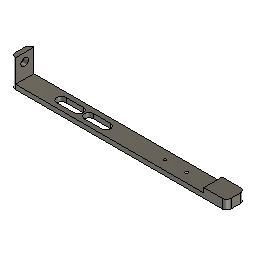
gearmotor winding v0 (Autodesk Fusion 360 design; units mm, degrees)
Autodesk Fusion 360 part; units mm, degrees
sketch "Sketch1" plane through (0, 0, 0) normal (0, 0, 1) x (1, 0, 0)
  line L0 (-70, 20) -> (165, 20)
  line L1 (165, 20) -> (165, 0)
  line L2 (165, 0) -> (-70, 0)
  line L3 (-70, 0) -> (-70, 20)
  dimension "d1" = 235
  dimension "d2" = 20
  constraint horizontal L0
  constraint vertical L1
  constraint horizontal L2
  constraint vertical L3
  measures "d1" distance of L0.start L0.end
  measures "d2" distance of L0.start L2.end
extrude "Extrude1" add sketch "Sketch1" along normal blind 5
sketch "Sketch2" plane through (0, 0, 5) normal (0, 0, 1) x (-1, 0, 0)
  line L0 (70, 0) -> (-165, 0)
  line L1 (-165, 0) -> (-165, -20)
  line L2 (-165, -20) -> (70, -20)
  line L3 (70, -20) -> (70, 0)
  circle A0 centre (-87.5581, -10.1163) radius 2.5
  circle A1 centre (-111.2788, -10.1163) radius 2.5
  line L4 (25.0313, -5.0352) -> (6.1177, -5.0352)
  arc A2 (6.1177, -5.0352) -> (6.1177, -15.0352) centre (6.1177, -10.0352) ccw
  line L5 (6.1177, -15.0352) -> (25.0313, -15.0352)
  arc A3 (25.0313, -15.0352) -> (25.0313, -5.0352) centre (25.0313, -10.0352) ccw
  line L6 (25.0313, -10.0352) -> (6.1177, -10.0352) construction
  line L7 (-5.3429, -4.8835) -> (-23.6696, -4.8835)
  arc A4 (-23.6696, -4.8835) -> (-23.6696, -14.8835) centre (-23.6696, -9.8835) ccw
  line L8 (-23.6696, -14.8835) -> (-5.3429, -14.8835)
  arc A5 (-5.3429, -14.8835) -> (-5.3429, -4.8835) centre (-5.3429, -9.8835) ccw
  line L9 (-5.3429, -9.8835) -> (-23.6696, -9.8835) construction
  point P0 (6.1177, -10.0352)
  dimension "d5" = 5
  dimension "d6" = 5
  dimension "d7" = 10
  dimension "d8" = 10
  constraint tangent L4 A2
  constraint tangent A2 L5
  constraint parallel L4 L5
  constraint tangent L5 A3
  constraint tangent L4 A3
  constraint parallel L2 L6
  constraint tangent L7 A4
  constraint tangent A4 L8
  constraint parallel L7 L8
  constraint tangent L8 A5
  constraint tangent L7 A5
  constraint parallel L5 L9
  measures "d5" diameter of A0
  measures "d6" diameter of A1
  measures "d7" diameter of A2
  measures "d8" diameter of A4
extrude "Extrude2" cut sketch "Sketch2" against normal blind 20 contours A0 | A1 | L4 A2 L5 A3 | L7 A4 L8 A5
fillet "Fillet1" radius 5 4 edges at (165, 0, 2.5) (165, 20, 2.5) (-70, 20, 2.5) (-70, 0, 2.5)
sketch "Sketch3" plane through (0, 0, 5) normal (0, 0, 1) x (-1, 0, 0)
  arc A0 (70, -5) -> (65, 0) centre (65, -5) ccw
  line L0 (65, 0) -> (-160, 0)
  arc A1 (-160, 0) -> (-165, -5) centre (-160, -5) ccw
  line L1 (-165, -5) -> (-165, -15)
  arc A2 (-165, -15) -> (-160, -20) centre (-160, -15) ccw
  line L2 (-160, -20) -> (65, -20)
  arc A3 (65, -20) -> (70, -15) centre (65, -15) ccw
  line L3 (70, -15) -> (70, -5)
  line L4 (6.1177, -5.0352) -> (25.0313, -5.0352)
  arc A4 (25.0313, -15.0352) -> (25.0313, -5.0352) centre (25.0313, -10.0352) ccw
  line L5 (25.0313, -15.0352) -> (6.1177, -15.0352)
  arc A5 (6.1177, -5.0352) -> (6.1177, -15.0352) centre (6.1177, -10.0352) ccw
  circle A6 centre (-111.2788, -10.1163) radius 2.5
  line L6 (-23.6696, -4.8835) -> (-5.3429, -4.8835)
  arc A7 (-5.3429, -14.8835) -> (-5.3429, -4.8835) centre (-5.3429, -9.8835) ccw
  line L7 (-5.3429, -14.8835) -> (-23.6696, -14.8835)
  arc A8 (-23.6696, -4.8835) -> (-23.6696, -14.8835) centre (-23.6696, -9.8835) ccw
  circle A9 centre (-87.5581, -10.1163) radius 2.5
  line L8 (-165, -20) -> (-140, -20)
  line L9 (-140, -20) -> (-140, 0)
  line L10 (-140, 0) -> (-165, 0)
  line L11 (-165, 0) -> (-165, -20)
  dimension "d13" = 25
  dimension "d14" = 20
  constraint horizontal L8
  constraint vertical L9
  constraint horizontal L10
  constraint vertical L11
  measures "d13" distance of L8.start L8.end
  measures "d14" distance of L8.start L10.end
extrude "Extrude3" add sketch "Sketch3" along normal blind 5 contours L0 A1 L1 A2 L2 L8 L9 L10 L11
sketch "Sketch4" plane through (0, 0, 5) normal (0, 0, 1) x (-1, 0, 0)
  line L0 (-140, 0) -> (-140, -20)
  line L1 (-140, -20) -> (65, -20)
  arc A0 (65, -20) -> (70, -15) centre (65, -15) ccw
  line L2 (70, -15) -> (70, -5)
  arc A1 (70, -5) -> (65, 0) centre (65, -5) ccw
  line L3 (65, 0) -> (-140, 0)
  line L4 (6.1177, -5.0352) -> (25.0313, -5.0352)
  arc A2 (25.0313, -15.0352) -> (25.0313, -5.0352) centre (25.0313, -10.0352) ccw
  line L5 (25.0313, -15.0352) -> (6.1177, -15.0352)
  arc A3 (6.1177, -5.0352) -> (6.1177, -15.0352) centre (6.1177, -10.0352) ccw
  circle A4 centre (-111.2788, -10.1163) radius 2.5
  line L6 (-23.6696, -4.8835) -> (-5.3429, -4.8835)
  arc A5 (-5.3429, -14.8835) -> (-5.3429, -4.8835) centre (-5.3429, -9.8835) ccw
  line L7 (-5.3429, -14.8835) -> (-23.6696, -14.8835)
  arc A6 (-23.6696, -4.8835) -> (-23.6696, -14.8835) centre (-23.6696, -9.8835) ccw
  circle A7 centre (-87.5581, -10.1163) radius 2.5
  line L8 (70, -20) -> (65, -20)
  line L9 (65, -20) -> (65, 0)
  line L10 (65, 0) -> (70, 0)
  line L11 (70, 0) -> (70, -20)
  dimension "d17" = 5
  dimension "d18" = 20
  constraint horizontal L8
  constraint vertical L9
  constraint horizontal L10
  constraint vertical L11
  measures "d17" distance of L8.start L1.end
  measures "d18" distance of L8.start L10.end
extrude "Extrude4" add sketch "Sketch4" along normal blind 25 contours A0 L2 A1 L9 L11
sketch "Sketch5" plane through (-65, 0, 0) normal (1, 0, 0) x (0, 1, 0)
  line L0 (0, 5) -> (20, 5)
  line L1 (20, 5) -> (20, 30)
  line L2 (20, 30) -> (0, 30)
  line L3 (0, 30) -> (0, 5)
  circle A0 centre (10, 21) radius 4.15
  dimension "d21" = 8.3
  dimension "d22" = 16
  measures "d21" diameter of A0
  measures "d22" distance of L0 A0.centre
extrude "Extrude5" cut sketch "Sketch5" against normal blind 6 contours A0
thread "Thread1" "ISO Metric profile 3.5 M3.5x0.6 6H" major diameter 3.5995 minor diameter 2.93 pitch 0.6 angle 60 resizes the face on face at (85.0705, 10.3652, 3.3333)
thread "Thread2" "ISO Metric profile 3.5 M3.5x0.6 6H" major diameter 3.5995 minor diameter 2.93 pitch 0.6 angle 60 resizes the face on face at (108.7912, 10.3652, 3.3333)
